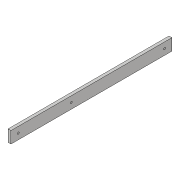
# Autodesk Inventor part: Needle Bearing Mount Connector 2
Saved by Autodesk Inventor 2018.3 (Build 223284000, 284)
## iProperties
Created: 2019-05-20
Part Number: Needle Bearing Mount Connector 2
Material: Generic
Document SubType Name: Modeling
Designer: aye06091
Mass: 7.02693 g
Surface Area: 56.8376 cm^2
Volume: 7.02693 cm^3
Density: 1 g/cm^3
Appearance: Default
Author: aye06091
Autodesk Inventor part; units mm, degrees
ref_plane "YZ Plane" through (0, 0, 0) normal (1, 0, 0) x (0, 1, 0)
ref_plane "XZ Plane" through (0, 0, 0) normal (0, 1, 0) x (-1, 0, 0)
ref_plane "XY Plane" through (0, 0, 0) normal (0, 0, 1) x (1, 0, 0)
sketch "Sketch1" plane through (0, 0, 0) normal (0, 0, 1) x (1, 0, 0)
  line L0 (0, 0) -> (3.175, 0)
  line L1 (3.175, 0) -> (3.175, -12.7)
  line L2 (3.175, -12.7) -> (0, -12.7)
  line L3 (0, -12.7) -> (0, 0)
  dimension "d0" = 12.7
  dimension "d1" = 3.175
  constraints: 8 end point, 2 parallel, 1 horizontal, 1 perpendicular
  measures "d0" distance of L0.end L1.end
  measures "d1" distance of L1.end L2.end
extrude "Extrusion1" add sketch "Sketch1" along normal blind 175.133
sketch "Sketch2" plane through (3.175, -12.7, 0) normal (1, 0, 0) x (0, 0, -1)
  line L0 (0, 12.7) -> (0, 0) projected
  circle A0 centre (-7.9375, 6.35) radius 0.7937
  circle A1 centre (-109.5375, 6.35) radius 0.7937
  circle A2 centre (-167.1955, 6.35) radius 0.7937
  dimension "d4" = 1.5875
  dimension "d5" = 7.9375
  dimension "d8" = 101.6
  dimension "d9" = 57.658
  dimension "d10" = 1.5875
  dimension "d11" = 1.5875
  constraints: 3 centre point
  measures "d4" diameter of A0
  measures "d5" distance from line of L0 A0.centre
  measures "d8" distance of A0.centre A1.centre
  measures "d9" distance of A1.centre A2.centre
  measures "d10" diameter of A1
  measures "d11" diameter of A2
extrude "Extrusion2" cut sketch "Sketch2" against normal blind 25.4
hole "Hole1" at (3.175, -6.35, 109.5375) direction (-1, 0, 0) diameter 2.159 end through all
hole "Hole2" at (3.175, -6.35, 167.1955) direction (-1, 0, 0) diameter 2.159 end through all
hole "Hole3" at (3.175, -6.35, 7.9375) direction (-1, 0, 0) diameter 2.159 end through all
body "Solid1"
